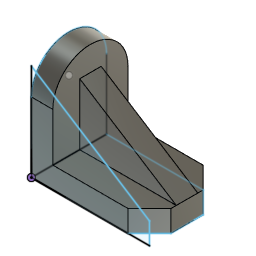
A1 (Autodesk Fusion 360 design; units mm, degrees)
Autodesk Fusion 360 part; units mm, degrees
sketch "back" plane through (0, 0, 0) normal (1, 0, 0) x (0, 1, 0)
  line L0 (0, 0) -> (42, 0)
  line L1 (0, 0) -> (0, 39)
  line L2 (42, 0) -> (42, 39)
  arc A0 (42, 39) -> (0, 39) centre (21, 39) ccw
  dimension "d1" = 42
  dimension "d3" = 39
  constraint coincident L0.start L1.start
  constraint horizontal L0
  constraint perpendicular L0 L1
  constraint perpendicular L0 L2
  constraint equal L1 L2
  measures "d1" distance of L0.start L0.end
  measures "d3" distance of L0.start L1.end
  measures "d9" distance of L0.start
extrude "Extrude1" add sketch "back" along normal blind 12 makes body 1
sketch "bottom" plane through (0, 0, 0) normal (0, 0, 1) x (1, 0, 0)
  line L0 (0, 0) -> (54, 0)
  line L1 (66, 12) -> (66, 30)
  line L2 (0, 0) -> (0, 42)
  line L3 (0, 42) -> (54, 42)
  line L4 (54, 42) -> (66, 30)
  line L5 (66, 12) -> (54, 0)
  dimension "d9" = 42
  constraint coincident L0.start L2.start
  constraint horizontal L0
  constraint perpendicular L0 L1
  constraint perpendicular L0 L2
  measures "d9" distance of L0.start L2.end
extrude "Extrude2" add sketch "bottom" along normal blind 12 separate body makes body 2
move_body "Move1" bodies 2 to x (1, 0, 0) y (0, 1, 0) z (0, 0, 1) at (0, -21, 0)
move_face "MoveFace1" by (0, -21, 0) 1 faces at (12, 14, 26) on bodies 1
move_body "Move2" bodies 1 to x (1, 0, 0) y (0, 1, 0) z (0, 0, 1) at (0, -21, 0)
sketch "middle" plane through (0, 0, 0) normal (0, 1, 0) x (1, 0, 0)
  line L0 (0, 0) -> (0, -54)
  line L1 (0, 0) -> (66, 0)
  line L2 (66, 0) -> (66, -12)
  line L3 (0, -54) -> (66, -12)
  dimension "d16" = 54
  dimension "d19" = 12
  constraint coincident L0.start L1.start
  constraint vertical L0
  constraint perpendicular L0 L1
  constraint perpendicular L1 L2
  measures "d16" distance of L0.start L0.end
  measures "d19" distance of L1.end L2.end
extrude "Extrude3" add sketch "middle" along normal mid plane 12 bodies 1 2
move_body "Move3" bodies 1 to x (1, 0, 0) y (0, 1, 0) z (0, 0, 1) at (0, 21, 0)
named bodies: "A1 piece", "bottom"
